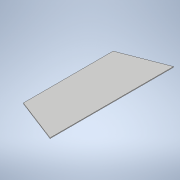
# Autodesk Inventor part: angledfloorfit
Saved by Autodesk Inventor 2021 (Build 250183000, 183)
## iProperties
Created: 2020-10-26
Part Number: angledfloorfit
Material: Generic
Document SubType Name: Modeling
Designer: mackeycj
Density: 1 g/cm^3
Appearance: Default
Author: mackeycj
Autodesk Inventor part; units mm, degrees
ref_plane "YZ Plane" through (0, 0, 0) normal (1, 0, 0) x (0, 1, 0)
ref_plane "XZ Plane" through (0, 0, 0) normal (0, 1, 0) x (-1, 0, 0)
ref_plane "XY Plane" through (0, 0, 0) normal (0, 0, 1) x (1, 0, 0)
sketch "Sketch1" plane through (0, 0, 0) normal (0, 1, 0) x (-1, 0, 0)
  line L0 (0, 0) -> (0, 279.4)
  line L1 (0, 0) -> (0, -279.4)
  line L2 (0, 0) -> (197.104, 0)
  line L3 (197.104, 0) -> (197.104, 203.2)
  line L4 (197.104, 0) -> (197.104, -203.2)
  line L5 (197.104, -203.2) -> (0, -279.4)
  line L6 (197.104, 203.2) -> (0, 279.4)
  dimension "d0" = 279.4
  dimension "d1" = 279.4
  dimension "d2" = 197.104
  dimension "d3" = 203.2
  dimension "d4" = 203.2
  constraints: 14 end point, 3 vertical, 1 horizontal, 1 perpendicular
  measures "d0" distance of L0.start L0.end
  measures "d1" distance of L0.start L1.end
  measures "d2" distance of L0.start L2.end
  measures "d3" distance of L2.end L3.end
  measures "d4" distance of L2.end L4.end
extrude "Extrusion1" add sketch "Sketch1" along normal blind 3.175
body "Solid1"
